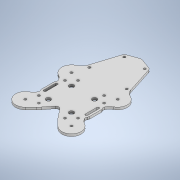
# Autodesk Inventor part: 399 prig z plate
Saved by Autodesk Inventor 2020 (Build 240168000, 168)
## iProperties
Created: 2022-05-23
Part Number: 399 prig z plate
Material: Generic
Document SubType Name: Modeling
Designer: Steven
Density: 1 g/cm^3
Appearance: Default
Author: Steven
Autodesk Inventor part; units mm, degrees
ref_plane "YZ Plane" through (0, 0, 0) normal (1, 0, 0) x (0, 1, 0)
ref_plane "XZ Plane" through (0, 0, 0) normal (0, 1, 0) x (-1, 0, 0)
ref_plane "XY Plane" through (0, 0, 0) normal (0, 0, 1) x (1, 0, 0)
sketch "Sketch1" plane through (0, 0, 0) normal (0, 1, 0) x (-1, 0, 0)
  arc A0 (-30.0072, 97.3212) -> (-35.8309, 103.5589) centre (-41.895, 92.0599) ccw
  arc A1 (-30.286, 94.3964) -> (-30.0072, 97.3212) centre (-32.7505, 96.107) ccw
  arc A2 (-30.286, 94.3964) -> (-31, 92.1156) centre (-27, 92.1156) ccw
  line L0 (-31, 92.1156) -> (-31, 77.1156)
  arc A3 (-31, 77.1156) -> (-30.286, 74.8348) centre (-27, 77.1156) ccw
  arc A4 (-30.0072, 71.9101) -> (-30.286, 74.8348) centre (-32.7505, 73.1242) ccw
  arc A5 (-35.8309, 65.6723) -> (-30.0072, 71.9101) centre (-41.895, 77.1713) ccw
  arc A6 (-35.8309, 65.6723) -> (-34.9925, 43.1559) centre (-30, 54.6156) ccw
  arc A7 (-27.7949, 35.1735) -> (-34.9925, 43.1559) centre (-40.1848, 31.2379) ccw
  line L1 (-27.7949, 35.1735) -> (-17.0958, 1.4913)
  arc A8 (-17.0958, 1.4913) -> (-14.6505, -1.0569) centre (-13.2835, 2.7022) ccw
  line L2 (-14.6505, -1.0569) -> (-2.0505, -5.6388)
  arc A9 (-2.0505, -5.6388) -> (2.0505, -5.6388) centre (0, 0) ccw
  line L3 (2.0505, -5.6388) -> (14.6505, -1.0569)
  arc A10 (14.6505, -1.0569) -> (17.0958, 1.4913) centre (13.2835, 2.7022) ccw
  line L4 (17.0958, 1.4913) -> (27.7949, 35.1735)
  arc A11 (34.9925, 43.1559) -> (27.7949, 35.1735) centre (40.1848, 31.2379) ccw
  arc A12 (34.9925, 43.1559) -> (35.8309, 65.6723) centre (30, 54.6156) ccw
  arc A13 (30.0072, 71.9101) -> (35.8309, 65.6723) centre (41.895, 77.1713) ccw
  arc A14 (30.286, 74.8348) -> (30.0072, 71.9101) centre (32.7505, 73.1242) ccw
  arc A15 (30.286, 74.8348) -> (31, 77.1156) centre (27, 77.1156) ccw
  line L5 (31, 77.1156) -> (31, 92.1156)
  arc A16 (31, 92.1156) -> (30.286, 94.3964) centre (27, 92.1156) ccw
  arc A17 (30.0072, 97.3212) -> (30.286, 94.3964) centre (32.7505, 96.107) ccw
  arc A18 (35.8309, 103.5589) -> (30.0072, 97.3212) centre (41.895, 92.0599) ccw
  arc A19 (35.8309, 103.5589) -> (21.1612, 123.4545) centre (30, 114.6156) ccw
  line L6 (21.1612, 123.4545) -> (13.9152, 116.2085)
  arc A20 (13.9152, 116.2085) -> (11.0366, 112.9476) centre (38.6639, 91.4597) ccw
  line L7 (11.0366, 112.9476) -> (3.1574, 102.8173)
  arc A21 (-3.1574, 102.8173) -> (3.1574, 102.8173) centre (0, 105.273) ccw
  line L8 (-3.1574, 102.8173) -> (-11.0366, 112.9476)
  arc A22 (-11.0366, 112.9476) -> (-13.9152, 116.2085) centre (-38.6639, 91.4597) ccw
  line L9 (-13.9152, 116.2085) -> (-21.1612, 123.4545)
  arc A23 (-21.1612, 123.4545) -> (-35.8309, 103.5589) centre (-30, 114.6156) ccw
  arc A24 (25.5, 77.1156) -> (28.5, 77.1156) centre (27, 77.1156) ccw
  line L10 (25.5, 92.1156) -> (25.5, 77.1156)
  arc A25 (28.5, 92.1156) -> (25.5, 92.1156) centre (27, 92.1156) ccw
  line L11 (28.5, 77.1156) -> (28.5, 92.1156)
  arc A26 (-28.5, 77.1156) -> (-25.5, 77.1156) centre (-27, 77.1156) ccw
  line L12 (-28.5, 92.1156) -> (-28.5, 77.1156)
  arc A27 (-25.5, 92.1156) -> (-28.5, 92.1156) centre (-27, 92.1156) ccw
  line L13 (-25.5, 77.1156) -> (-25.5, 92.1156)
  circle A28 centre (-30, 54.6156) radius 1.5
  circle A29 centre (-13.2835, 2.7022) radius 1.5
  circle A30 centre (-25.4558, 101.5862) radius 1.5
  circle A31 centre (-25.4558, 67.6451) radius 1.5
  circle A32 centre (-15, 99.6156) radius 3
  circle A33 centre (25.4558, 67.6451) radius 1.5
  circle A34 centre (25.4558, 101.5862) radius 1.5
  circle A35 centre (15, 69.6156) radius 3
  circle A36 centre (30, 54.6156) radius 1.5
  circle A37 centre (30, 114.6156) radius 1.5
  circle A38 centre (24.2029, 37.0782) radius 1.5
  circle A39 centre (13.2835, 2.7022) radius 1.5
  circle A40 centre (16.9706, 110.0715) radius 1.5
  circle A41 centre (16.9706, 59.1598) radius 1.5
  circle A42 centre (15, 99.6156) radius 3
  circle A43 centre (-15, 69.6156) radius 3
  circle A44 centre (-16.9706, 59.1598) radius 1.5
  circle A45 centre (-16.9706, 110.0715) radius 1.5
  circle A46 centre (-24.2029, 37.0782) radius 1.5
  circle A47 centre (-30, 114.6156) radius 1.5
  point P0 (-30.286, 94.3964)
  point P1 (-35.8309, 65.6723)
  point P2 (-34.9925, 43.1559)
  point P3 (-27.7949, 35.1735)
  point P4 (-17.0958, 1.4913)
  point P5 (-14.6505, -1.0569)
  point P6 (2.0505, -5.6388)
  point P7 (14.6505, -1.0569)
  point P8 (27.7949, 35.1735)
  point P9 (35.8309, 65.6723)
  point P10 (30.0072, 71.9101)
  point P11 (30.286, 74.8348)
  point P12 (30.286, 94.3964)
  point P13 (30.0072, 97.3212)
  point P14 (13.9152, 116.2085)
  point P15 (11.0366, 112.9476)
  point P16 (-3.1574, 102.8173)
  point P17 (-13.9152, 116.2085)
  point P18 (-21.1612, 123.4545)
  point P19 (-35.8309, 103.5589)
  point P20 (-30.0072, 97.3212)
  point P21 (25.5, 77.1156)
  point P22 (28.5, 77.1156)
  constraints: 56 point on circle, 48 centre point, 28 end point
extrude "Extrusion1" add sketch "Sketch1" along normal blind 3
sketch "Sketch2" plane through (0, 3, 0) normal (0, 1, 0) x (1, 0, 0)
  line L0 (31, -92.1156) -> (31, -77.1156) construction
  arc A0 (31, -77.1156) -> (30.286, -74.8348) centre (27, -77.1156) ccw construction
  arc A1 (30.0072, -71.9101) -> (30.286, -74.8348) centre (32.7505, -73.1242) ccw construction
  arc A2 (35.8309, -65.6723) -> (30.0072, -71.9101) centre (41.895, -77.1713) ccw construction
  arc A3 (35.8309, -65.6723) -> (34.9925, -43.1559) centre (30, -54.6156) ccw construction
  arc A4 (27.7949, -35.1735) -> (34.9925, -43.1559) centre (40.1848, -31.2379) ccw construction
  line L1 (27.7949, -35.1735) -> (17.0958, -1.4913) construction
  arc A5 (17.0958, -1.4913) -> (14.6505, 1.0569) centre (13.2835, -2.7022) ccw construction
  line L2 (14.6505, 1.0569) -> (2.0505, 5.6388) construction
  arc A6 (2.0505, 5.6388) -> (-2.0505, 5.6388) centre (0, 0) ccw construction
  line L3 (-2.0505, 5.6388) -> (-14.6505, 1.0569) construction
  arc A7 (-14.6505, 1.0569) -> (-17.0958, -1.4913) centre (-13.2835, -2.7022) ccw construction
  line L4 (-17.0958, -1.4913) -> (-27.7949, -35.1735) construction
  arc A8 (-34.9925, -43.1559) -> (-27.7949, -35.1735) centre (-40.1848, -31.2379) ccw construction
  arc A9 (-34.9925, -43.1559) -> (-35.8309, -65.6723) centre (-30, -54.6156) ccw construction
  arc A10 (-30.0072, -71.9101) -> (-35.8309, -65.6723) centre (-41.895, -77.1713) ccw construction
  arc A11 (-30.286, -74.8348) -> (-30.0072, -71.9101) centre (-32.7505, -73.1242) ccw construction
  arc A12 (-30.286, -74.8348) -> (-31, -77.1156) centre (-27, -77.1156) ccw construction
  line L5 (-31, -77.1156) -> (-31, -92.1156) construction
  arc A13 (-31, -92.1156) -> (-30.286, -94.3964) centre (-27, -92.1156) ccw construction
  arc A14 (-30.0072, -97.3212) -> (-30.286, -94.3964) centre (-32.7505, -96.107) ccw construction
  arc A15 (-35.8309, -103.5589) -> (-30.0072, -97.3212) centre (-41.895, -92.0599) ccw construction
  arc A16 (-35.8309, -103.5589) -> (-21.1612, -123.4545) centre (-30, -114.6156) ccw construction
  line L6 (-21.1612, -123.4545) -> (-13.9152, -116.2085) construction
  arc A17 (-13.9152, -116.2085) -> (-11.0366, -112.9476) centre (-38.6639, -91.4597) ccw construction
  line L7 (-11.0366, -112.9476) -> (-3.1574, -102.8173) construction
  arc A18 (3.1574, -102.8173) -> (-3.1574, -102.8173) centre (0, -105.273) ccw construction
  line L8 (3.1574, -102.8173) -> (11.0366, -112.9476) construction
  arc A19 (11.0366, -112.9476) -> (13.9152, -116.2085) centre (38.6639, -91.4597) ccw construction
  line L9 (13.9152, -116.2085) -> (21.1612, -123.4545) construction
  arc A20 (21.1612, -123.4545) -> (35.8309, -103.5589) centre (30, -114.6156) ccw construction
  arc A21 (30.0072, -97.3212) -> (35.8309, -103.5589) centre (41.895, -92.0599) ccw construction
  arc A22 (30.286, -94.3964) -> (30.0072, -97.3212) centre (32.7505, -96.107) ccw construction
  arc A23 (30.286, -94.3964) -> (31, -92.1156) centre (27, -92.1156) ccw construction
  circle A24 centre (25.4558, -101.5862) radius 1.5 construction
  circle A25 centre (-16.9706, -110.0715) radius 1.5 projected
  circle A26 centre (-15, -99.6156) radius 3 construction
  circle A27 centre (-15, -69.6156) radius 3 construction
  circle A28 centre (-24.2029, -37.0782) radius 1.5 construction
  circle A29 centre (24.2029, -37.0782) radius 1.5 construction
  circle A30 centre (15, -69.6156) radius 3 construction
  circle A31 centre (16.9706, -59.1598) radius 1.5 construction
  circle A32 centre (30, -54.6156) radius 1.5 construction
  circle A33 centre (25.4558, -67.6451) radius 1.5 construction
  circle A34 centre (16.9706, -110.0715) radius 1.5 projected
  circle A35 centre (15, -99.6156) radius 3 construction
  circle A36 centre (-25.4558, -67.6451) radius 1.5 construction
  circle A37 centre (-16.9706, -59.1598) radius 1.5 construction
  circle A38 centre (-25.4558, -101.5862) radius 1.5 construction
  circle A39 centre (-30, -54.6156) radius 1.5 construction
  circle A40 centre (-13.2835, -2.7022) radius 1.5 construction
  circle A41 centre (13.2835, -2.7022) radius 1.5 construction
  circle A42 centre (30, -114.6156) radius 1.5 projected
  line L10 (-25.5, -77.1156) -> (-25.5, -92.1156) construction
  arc A43 (-28.5, -92.1156) -> (-25.5, -92.1156) centre (-27, -92.1156) ccw construction
  line L11 (-28.5, -92.1156) -> (-28.5, -77.1156) construction
  arc A44 (-25.5, -77.1156) -> (-28.5, -77.1156) centre (-27, -77.1156) ccw construction
  circle A45 centre (-30, -114.6156) radius 1.5 projected
  line L12 (28.5, -77.1156) -> (28.5, -92.1156) construction
  arc A46 (25.5, -92.1156) -> (28.5, -92.1156) centre (27, -92.1156) ccw construction
  line L13 (25.5, -92.1156) -> (25.5, -77.1156) construction
  arc A47 (28.5, -77.1156) -> (25.5, -77.1156) centre (27, -77.1156) ccw construction
  circle A48 centre (16.9706, -110.0715) radius 5 construction
  circle A49 centre (-16.9706, -110.0715) radius 5 construction
  arc A50 (-31.1155, -107.199) -> (-30, -122.1156) centre (-30, -114.6156) ccw
  arc A51 (30, -122.1156) -> (31.1155, -107.199) centre (30, -114.6156) ccw
  line L14 (30, -122.1156) -> (-30, -122.1156)
  line L15 (-16.9706, -105.0715) -> (16.9706, -105.0715)
  line L16 (-16.9706, -105.0715) -> (-31.1155, -107.199)
  line L17 (16.9706, -105.0715) -> (31.1155, -107.199)
  arc A52 (31.1155, -107.199) -> (30, -122.1156) centre (30, -114.6156) ccw construction
  arc A53 (-30, -122.1156) -> (-31.1155, -107.199) centre (-30, -114.6156) ccw construction
  line L18 (0, -105.273) -> (0, -113.6943) construction
  line L19 (0, -113.6943) -> (3.1574, -113.6943) construction
  line L20 (0, -113.6943) -> (0, -122.1156) construction
  circle A54 centre (0, -109.4837) radius 1.55
  line L21 (0, -117.905) -> (15.6117, -117.905) construction
  line L22 (13.9152, -116.2085) -> (21.1612, -123.4545) projected
  line L23 (0, -117.905) -> (-15.6117, -117.905) construction
  line L24 (-21.1612, -123.4545) -> (-13.9152, -116.2085) projected
  circle A55 centre (7.8058, -117.905) radius 1.55
  circle A56 centre (-7.8058, -117.905) radius 1.55
  dimension "d2" = 10
  dimension "d3" = 10
  dimension "d4" = 15
  dimension "d5" = 15
  dimension "d8" = 3.1
  dimension "d9" = 3.1
  dimension "d10" = 3.1
  constraints: 18 end point, 8 point on circle, 7 centre point, 5 midpoint, 4 coincident, 4 horizontal, 3 point on line, 3 tangent, 2 vertical alignment, 4 other
  measures "d4" diameter of A50
  measures "d5" diameter of A51
  measures "d8" diameter of A54
  measures "d9" diameter of A55
  measures "d10" diameter of A56
extrude "Extrusion2" [suppressed]
body "Solid1"
